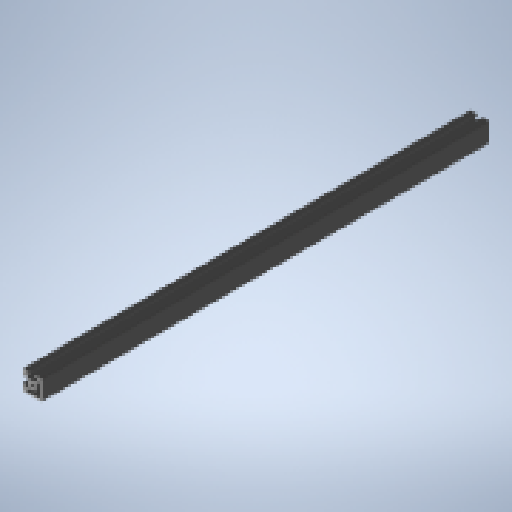
# Autodesk Inventor part: HFSTB5-2020-456
Saved by Autodesk Inventor 2024 (Build 280153000, 153)
## iProperties
Category: PARTsolutions
Company: MISUMI
Created: 2024-08-20
Part Number: HFSTB5-2020-456
Material: Aluminum 6061
Catalog Web Link: www.cadenas.de
Description: NFS5-2020, NFSB5-2020, HFS5-2020, HFSB5-2020, CAF5-2020, HFSY5-2020, NFSF5-2020, HFSF5-2020, HFSFB5-2020, NFST5-2020, HFST5-2020, HFSTB5-2020, HFSH5-2020, HFSC5-2020-HFS5 Series Aluminum Extrusions 20 Square -1 Slot-
Vendor: MISUMI
Document SubType Name: Modeling
Designer: psAdmin
Manufacturer: MISUMI
Mass: 240.688 g
Surface Area: 837.523 cm^2
Volume: 89.1436 cm^3
Density: 2.7 g/cm^3
Appearance: Aluminum - Flat
PSOL_IDENT_0: {$CADENAS_DATA/23d-libs/misumi/metric/38_al_extrusions_blackets/5/hfs5_2020.prj},681 {VTYP=3D},{NB=H
PSOL_IDENT_1: FSTB5-2020-456},{LINA=HFSTB5-2020-456},{NN=NFS5-2020, NFSB5-2020, HFS5-2020, HFSB5-2020, CAF5-2020,
PSOL_IDENT_2: HFSY5-2020, NFSF5-2020, HFSF5-2020, HFSFB5-2020, NFST5-2020, HFST5-2020, HFSTB5-2020, HFSH5-2020, HF
PSOL_IDENT_3: SC5-2020},{DATE=08.05.2023 08:39:06},{GEOMDATE=27.07.2021 03:20:00},{VERSION=},{LINEID=110},{WBVAR=L
PSOL_IDENT_4: ,ALT1,ALT2,ALT4,ALT5,CP5,DL5,DR5,ALT6,ALT9,ALT10,ALT11,HP6,NHL6,DL6,NHR6,DR6,ALT7,ALT8,NH9,AH,BH,CH,
PSOL_IDENT_5: DH,EH,NH10,AV,BV,CV,DV,EV,NH11,AP,BP,CP,DP,EP,ALT12,ALT13,Z,NH12,XA,XB,XC,XD,XE,NH13,YA,YB,YC,YD,YE,
PSOL_IDENT_6: ALT16,HP16,DL16,DR16,ALT17,HQ17,JLP,ALT20},{WBNUMERIC=L,NH9,AH,BH,CH,DH,EH,NH10,AV,BV,CV,DV,EV,NH11,
PSOL_IDENT_7: AP,BP,CP,DP,EP,NH12,XA,XB,XC,XD,XE,NH13,YA,YB,YC,YD,YE,HQ17,JLP}  {NB=HFSTB5-2020-456},{LINA=HFSTB5-
PSOL_IDENT_8: 2020-456},{KT=DUMMY},{PN=HFSTB5-2020-456},{TPS=HFSTB5-2020},{MAT=A6N01SS-T5 Aluminum Alloy or 6005A-
PSOL_IDENT_9: T5 Aluminum Alloy},{ST=Black Anodize},{FRMW=20},{FRMH=20},{FRD=4.2},{L=456},{MASS=0.53},{SA=196},{LX=
PSOL_IDENT_10: 0.808x10^4},{LY=0.808x10^4},{ALT1=},{M1=0},{DPL1=0},{DPR1=0},{ALT1PN=},{ALT2=},{ALT2ALG= '','w/o End
PSOL_IDENT_11: Tapping (Heli-Coil Insert)','LHP','with LHP (Tapping on the Left (Heli-Coil Insert))','RHP','with R
PSOL_IDENT_12: HP (Tapping on the Right (Heli-Coil Insert))','HPW','with HPW (Tapping on Both Ends (Heli-Coil Inser
PSOL_IDENT_13: t))' },{M2=0},{DP2=0},{ALT2PN=},{ALT4=},{ALT4ALG= '', 'w/o SC (High Precision Cut)', 'SC', 'with SC
PSOL_IDENT_14: (High Precision Cut)' },{ALT4PN=},{ALT5=},{ALT5ALG= '','w/o 45 Degree Cut','1','with 45 Degree Cut'
PSOL_IDENT_15: },{CP5=},{CP5ALG= '','N/A' },{DL5=},{DL5ALG= '','N/A' },{DR5=},{DR5ALG= '','N/A' },{FRMLALT5=0},{FRM
PSOL_IDENT_16: RALT5=0},{ALT5PN=},{ALT6=},{ALT6ALG= '','w/o Fastening Location Wrench Access Hole Alterations','1','
PSOL_IDENT_17: with Fastening Location Wrench Access Hole Alterations' },{ALT9=},{ALT9ALG= '','w/o Location Specifi
PSOL_IDENT_18: ed Wrench Access Hole Alteratons (Horizontal)','1','with Location Specified Wrench Access Hole Alter
PSOL_IDENT_19: atons (Horizontal)' },{ALT10=},{ALT10ALG= '','w/o Location Specified Wrench Access Hole Alteratons (
PSOL_IDENT_20: Vertical)','1','with Location Specified Wrench Access Hole Alteratons (Vertical)' },{ALT11=},{ALT11A
PSOL_IDENT_21: LG= '','w/o Location Specified Wrench Access Hole Alteratons (Crisscross)','1','with Location Specif
PSOL_IDENT_22: ied Wrench Access Hole Alteratons (Crisscross)' },{HP6=},{HP6ALG= '','N/A' },{NHL6=},{NHL6ALG= '','N
PSOL_IDENT_23: /A' },{DL6=},{DL6ALG= '','N/A' },{NHR6=},{NHR6ALG= '','N/A' },{DR6=},{DR6ALG= '','N/A' },{HL6=0.000}
PSOL_IDENT_24: ,{HL6D=0},{HR6=0.000},{HR6D=0},{J6=0},{J6D=0},{K6=0},{K6D=0},{DD6=0.00},{DD6ALG=0},{ALT7=},{ALT7ALG=
PSOL_IDENT_25: '','N/A' },{ALT8=},{ALT8ALG= '','N/A' },{ALT678PN=},{NH9=0},{NH9MAX=5},{NH9ALG=[0]},{AH=0.0},{AHMIN=
PSOL_IDENT_26: 7},{AHMAX=451},{AHALG=[0]},{BH=0.0},{BHMIN=2},{BHMAX=453},{BHALG=[0]},{CH=0.0},{CHMIN=2},{CHMAX=455}
PSOL_IDENT_27: ,{CHALG=[0]},{DH=0.0},{DHMIN=2},{DHMAX=457},{DHALG=[0]},{EH=0.0},{EHMIN=2},{EHMAX=449},{EHALG=[0]},{
PSOL_IDENT_28: NH10=0},{NH10MAX=5},{NH10ALG=[0]},{AV=0.0},{AVMIN=7},{AVMAX=451},{AVALG=[0]},{BV=0.0},{BVMIN=2},{BVM
PSOL_IDENT_29: AX=453},{BVALG=[0]},{CV=0.0},{CVMIN=2},{CVMAX=455},{CVALG=[0]},{DV=0.0},{DVMIN=2},{DVMAX=457},{DVALG=
PSOL_IDENT_30: [0]},{EV=0.0},{EVMIN=2},{EVMAX=449},{EVALG=[0]},{NH11=0},{NH11MAX=5},{NH11ALG=[0]},{AP=0.0},{APMIN=7
PSOL_IDENT_31: },{APMAX=451},{APALG=[0]},{BP=0.0},{BPMIN=2},{BPMAX=453},{BPALG=[0]},{CP=0.0},{CPMIN=2},{CPMAX=455},
PSOL_IDENT_32: {CPALG=[0]},{DP=0.0},{DPMIN=2},{DPMAX=457},{DPALG=[0]},{EP=0.0},{EPMIN=2},{EPMAX=449},{EPALG=[0]},{A
PSOL_IDENT_33: LT9PN=},{ALT10PN=},{ALT11PN=},{ALT91011PN=},{ALT12=},{ALT12ALG= '','w/o Counterbore Hole in Specifie
PSOL_IDENT_34: d Position (Vertical)','1','with Counterbore Hole in Specified Position (Vertical)' },{ALT13=},{ALT1
PSOL_IDENT_35: 3ALG= '','N/A' },{Z=},{ZALG= '','N/A' },{DD12=0.0},{DD112=0.0},{NH12=0},{NH12MAX=5},{NH12ALG=[0]},{X
PSOL_IDENT_36: A=0.0},{XAMIN=7},{XAMAX=451},{XAALG=[0]},{XB=0.0},{XBMIN=2},{XBMAX=453},{XBALG=[0]},{XC=0.0},{XCMIN=
PSOL_IDENT_37: 2},{XCMAX=455},{XCALG=[0]},{XD=0.0},{XDMIN=2},{XDMAX=457},{XDALG=[0]},{XE=0.0},{XEMIN=2},{XEMAX=449}
PSOL_IDENT_38: ,{XEALG=[0]},{NH13=0},{NH13MAX=5},{NH13ALG=[0]},{YA=0.0},{YAMIN=7},{YAMAX=451},{YAALG=[0]},{YB=0.0},
PSOL_IDENT_39: {YBMIN=2},{YBMAX=453},{YBALG=[0]},{YC=0.0},{YCMIN=2},{YCMAX=455},{YCALG=[0]},{YD=0.0},{YDMIN=2},{YDM
PSOL_IDENT_40: AX=457},{YDALG=[0]},{YE=0.0},{YEMIN=2},{YEMAX=449},{YEALG=[0]},{ALT12PN=},{ALT13PN=},{ALT1213PN=},{A
PSOL_IDENT_41: LT16=},{ALT16ALG= '','w/o M Type Hole Alteration','1','with M Type Hole Alteration' },{HP16=},{HP16A
PSOL_IDENT_42: LG= '','N/A' },{DL16=},{DL16ALG= '','N/A' },{DR16=},{DR16ALG= '','N/A' },{H116=0},{D16=0.0},{ALT16PN=
PSOL_IDENT_43: },{ALT17=},{ALT17ALG= '','w/o L Type Hole Alteration (Top)','1','with L Type Hole Alteration (Top)'
PSOL_IDENT_44: },{HQ17=0},{HQ17ALG=0},{JLP=0},{JLPMIN=4.9},{JLPMAX=0},{JLPALG=[0]},{L17=0},{D17=0.0},{ALT17PN=},{AL
PSOL_IDENT_45: T20=},{ALT20PN=},{ERRORALT01=OK},{ERRORALT02=OK},{ERRORALT05=OK},{ERRORALT06091=OK},{ERRORALT06092=O
PSOL_IDENT_46: K},{ERRORALT06093=OK},{ERRORALT06094=OK},{ERRORALT06101=OK},{ERRORALT06102=OK},{ERRORALT06103=OK},{E
PSOL_IDENT_47: RRORALT06104=OK},{ERRORALT06111=OK},{ERRORALT06112=OK},{ERRORALT06113=OK},{ERRORALT06114=OK},{ERRORA
PSOL_IDENT_48: LT06121=OK},{ERRORALT06122=OK},{ERRORALT06123=OK},{ERRORALT06124=OK},{ERRORALT06131=OK},{ERRORALT061
PSOL_IDENT_49: 32=OK},{ERRORALT06133=OK},{ERRORALT06134=OK},{ERRORALT0616=OK},{ERRORALT06171=OK},{ERRORALT06172=OK}
PSOL_IDENT_50: ,{ERRORALT06173=OK},{ERRORALT0911=OK},{ERRORALT0913=OK},{ERRORALT0916=OK},{ERRORALT0917=OK},{ERRORAL
PSOL_IDENT_51: T1011=OK},{ERRORALT1012=OK},{ERRORALT1016=OK},{ERRORALT1017=OK},{ERRORALT1112=OK},{ERRORALT1113=OK},
PSOL_IDENT_52: {ERRORALT1116=OK},{ERRORALT1117=OK},{ERRORALT1216=OK},{ERRORALT1217=OK},{ERRORALT1316=OK},{ERRORALT1
PSOL_IDENT_53: 317=OK},{ERRORALT1617=OK},{ERRORPN=},{TFW=5}
NB: HFSTB5-2020-456
NN: NFS5-2020, NFSB5-2020, HFS5-2020, HFSB5-2020, CAF5-2020, HFSY5-2020, NFSF5-2020, HFSF5-2020, HFSFB5-2020, NFST5-2020, HFST5-2020, HFSTB5-2020, HFSH5-2020, HFSC5-2020
NT: HFS5 Series Aluminum Extrusions 20 Square -1 Slot-
NBSYN: $PN.
LINA: HFSTB5-2020-456
CATALOG: Misumi
PN: HFSTB5-2020-456
TPS: HFSTB5-2020
MAT: A6N01SS-T5 Aluminum Alloy or 6005A-T5 Aluminum Alloy
ST: Black Anodize
L: 456
MASS: 0.53
SA: 196
LX: 0.808x10^4
LY: 0.808x10^4
ALT1: w/o End Tapping
M1: 0
DPL1: 0
DPR1: 0
ALT2: w/o End Tapping (Heli-Coil Insert)
M2: 0
DP2: 0
ALT4: w/o SC (High Precision Cut)
ALT5: w/o 45 Degree Cut
CP5: N/A
DL5: N/A
DR5: N/A
ALT6: w/o Fastening Location Wrench Access Hole Alterations
ALT9: w/o Location Specified Wrench Access Hole Alteratons (Horizontal)
ALT10: w/o Location Specified Wrench Access Hole Alteratons (Vertical)
ALT11: w/o Location Specified Wrench Access Hole Alteratons (Crisscross)
HP6: N/A
NHL6: N/A
DL6: N/A
NHR6: N/A
DR6: N/A
HL6D: 0
HR6D: 0
J6D: 0
K6D: 0
DD6: 0
ALT7: N/A
ALT8: N/A
NH9: 0
AH: 0
BH: 0
CH: 0
DH: 0
EH: 0
NH10: 0
AV: 0
BV: 0
CV: 0
DV: 0
EV: 0
NH11: 0
AP: 0
BP: 0
CP: 0
DP: 0
EP: 0
ALT12: w/o Counterbore Hole in Specified Position (Vertical)
ALT13: N/A
Z: N/A
DD12: 0
DD112: 0
NH12: 0
XA: 0
XB: 0
XC: 0
XD: 0
XE: 0
NH13: 0
YA: 0
YB: 0
YC: 0
YD: 0
YE: 0
ALT16: w/o M Type Hole Alteration
HP16: N/A
DL16: N/A
DR16: N/A
H116: 0
D16: 0
ALT17: w/o L Type Hole Alteration (Top)
HQ17: 0
JLP: 0
D17: 0
ALT20: w/o CW (End Face C Chamfering)
SUPPLIER: MISUMI
ARTICLENO: HFSTB5-2020-456
BOMINFO: HFSTB5-2020-456
CREATOR: CADENAS GmbH
Title: HFSTB5-2020-456
Author: Cadenas PARTsolutions
Comments: HFS5 Series Aluminum Extrusions 20 Square -1 Slot-
Autodesk Inventor part; units mm, degrees
sketch "Sketch_64" plane through (0, 0, 0) normal (0, 0, 1) x (1, 0, 0)
  line L0 (-10, -3) -> (-10, -9)
  arc A0 (-10, -9) -> (-9, -10) centre (-9, -9) ccw
  line L1 (-9, -10) -> (9, -10)
  arc A1 (9, -10) -> (10, -9) centre (9, -9) ccw
  line L2 (10, -9) -> (10, 9)
  arc A2 (10, 9) -> (9, 10) centre (9, 9) ccw
  line L3 (9, 10) -> (3, 10)
  line L4 (3, 10) -> (3, 8)
  line L5 (3, 8) -> (6, 8)
  line L6 (6, 8) -> (6, 7.0607)
  line L7 (6, 7.0607) -> (2.9393, 4)
  line L8 (2.9393, 4) -> (0.5196, 4)
  line L9 (0.5196, 4) -> (0, 3.7)
  line L10 (0, 3.7) -> (-0.5196, 4)
  line L11 (-0.5196, 4) -> (-2.9393, 4)
  line L12 (-2.9393, 4) -> (-6, 7.0607)
  line L13 (-6, 7.0607) -> (-6, 8)
  line L14 (-6, 8) -> (-3, 8)
  line L15 (-3, 8) -> (-3, 10)
  line L16 (-3, 10) -> (-9, 10)
  arc A3 (-9, 10) -> (-10, 9) centre (-9, 9) ccw
  line L17 (-10, 9) -> (-10, 3)
  line L18 (-10, 3) -> (-8, 3)
  line L19 (-8, 3) -> (-8, 6)
  line L20 (-8, 6) -> (-7.0607, 6)
  line L21 (-7.0607, 6) -> (-4, 2.9393)
  line L22 (-4, 2.9393) -> (-4, 0.5196)
  line L23 (-4, 0.5196) -> (-3.7, 0)
  line L24 (-3.7, 0) -> (-4, -0.5196)
  line L25 (-4, -0.5196) -> (-4, -2.9393)
  line L26 (-4, -2.9393) -> (-7.0607, -6)
  line L27 (-7.0607, -6) -> (-8, -6)
  line L28 (-8, -6) -> (-8, -3)
  line L29 (-8, -3) -> (-10, -3)
  line L30 (-6, -7.2678) -> (-6, -7.5)
  arc A4 (-6, -7.5) -> (-5.5, -8) centre (-5.5, -7.5) ccw
  line L31 (-5.5, -8) -> (7, -8)
  arc A5 (7, -8) -> (8, -7) centre (7, -7) ccw
  line L32 (8, -7) -> (8, 5.5)
  arc A6 (8, 5.5) -> (7.5, 6) centre (7.5, 5.5) ccw
  line L33 (7.5, 6) -> (7.2678, 6)
  arc A7 (7.2678, 6) -> (6.9142, 5.8536) centre (7.2678, 5.5) ccw
  line L34 (6.9142, 5.8536) -> (4.1464, 3.0858)
  arc A8 (4.1464, 3.0858) -> (4, 2.7322) centre (4.5, 2.7322) ccw
  line L35 (4, 2.7322) -> (4, -1)
  arc A9 (1, -4) -> (4, -1) centre (1, -1) ccw
  line L36 (1, -4) -> (-2.7322, -4)
  arc A10 (-2.7322, -4) -> (-3.0858, -4.1464) centre (-2.7322, -4.5) ccw
  line L37 (-3.0858, -4.1464) -> (-5.8536, -6.9142)
  arc A11 (-5.8536, -6.9142) -> (-6, -7.2678) centre (-5.5, -7.2678) ccw
  constraints: 76 end point, 24 point on circle, 12 centre point
extrude "Extrusion1" add sketch "Sketch_64" against normal blind 456
sketch "Sketch2" plane through (0, 0, -456) normal (0, 0, -1) x (-1, 0, 0)
  point P0 (0, 0)
hole "Hole1" at (0, 0, -456) direction (0, 0, 1) diameter 4.2 depth 456
ref_plane "C1_XY" through (0, 0, 0) normal (0, 0, 1) x (1, 0, 0)
ref_plane "C1_YZ" through (0, 0, 0) normal (1, 0, 0) x (0, 1, 0)
ref_plane "C1_ZX" through (0, 0, 0) normal (0, 1, 0) x (0, 0, 1)
thread "Thread1" size "M5x0.8" class "6H" standard "ANSI Metric M Profile" length 10
thread "Thread2" size "M4.5x0.75" class "6H" standard "ANSI Metric M Profile" length 10
body "Solid1"
